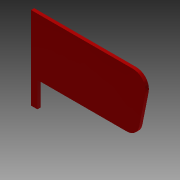
# Autodesk Inventor part: ImprintPart1
Saved by Autodesk Inventor 2014 Beta1 (Build 180079000, 79) ContinuousBuild 0
## iProperties
Created: 2012-10-22
Part Number: ImprintPart1
Material: Generic
Document SubType Name: Modeling
Designer: ekinsb
Density: 1 g/cm^3
Appearance: Smooth - Red
Author: ekinsb
Autodesk Inventor part; units mm, degrees
ref_plane "YZ Plane" through (0, 0, 0) normal (1, 0, 0) x (0, 1, 0)
ref_plane "XZ Plane" through (0, 0, 0) normal (0, 1, 0) x (-1, 0, 0)
ref_plane "XY Plane" through (0, 0, 0) normal (0, 0, 1) x (1, 0, 0)
sketch "Sketch1" plane through (0, 0, 0) normal (0, 0, 1) x (1, 0, 0)
  line L0 (0, 0) -> (190.5, 0)
  arc A0 (190.5, 0) -> (215.4067, 20.4187) centre (190.5, 25.4) ccw
  line L1 (215.4067, 20.4187) -> (228.1067, 83.9187)
  arc A1 (228.1067, 83.9187) -> (203.2, 114.3) centre (203.2, 88.9) ccw
  line L2 (203.2, 114.3) -> (0, 114.3)
  line L3 (0, 114.3) -> (0, 0)
  dimension "d4" = 25.4
  dimension "d5" = 25.4
  dimension "d6" = 228.6
  dimension "d9" = 114.3
  constraints: 8 end point, 4 point on circle, 4 tangent, 2 centre point, 1 coincident
  measures "d4" radius of A1
  measures "d5" radius of A0
  measures "d9" distance of L2.end L0.start
extrude "Extrusion1" add sketch "Sketch1" along normal blind 6.35
body "Solid1"
